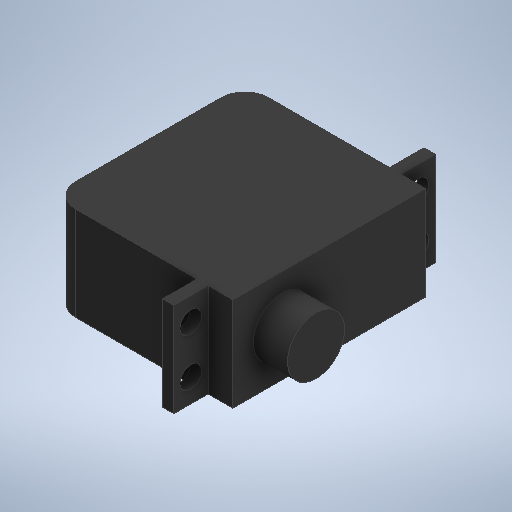
# Autodesk Inventor part: servomoteur_roues
Saved by Autodesk Inventor 2025 (Build 290162000, 162)
## iProperties
Created: 2024-09-04
Part Number: servomoteur_roues
Material: Générique
Document SubType Name: Modeling
Designer: chass
Density: 1 g/cm^3
Appearance: Par défaut
Author: chass
Autodesk Inventor part; units mm, degrees
ref_plane "YZ Plane" through (0, 0, 0) normal (1, 0, 0) x (0, 1, 0)
ref_plane "XZ Plane" through (0, 0, 0) normal (0, 1, 0) x (-1, 0, 0)
ref_plane "XY Plane" through (0, 0, 0) normal (0, 0, 1) x (1, 0, 0)
sketch "Esquisse1" plane through (0, 0, 0) normal (1, 0, 0) x (0, 1, 0)
  line L0 (9.85, 20.25) -> (-9.85, 20.25)
  line L1 (-9.85, 20.25) -> (-9.85, -20.25)
  line L2 (-9.85, -20.25) -> (9.85, -20.25)
  line L3 (9.85, -20.25) -> (9.85, 20.25)
  line L4 (9.85, 20.25) -> (-9.85, -20.25)
  line L5 (-9.85, 20.25) -> (9.85, -20.25)
  point P0 (0, 0)
  point P1 (0, 0)
  point P2 (0, 0)
  dimension "d0" = 19.7
  dimension "d1" = 40.5
  constraints: 12 end point, 2 midpoint, 2 parallel, 1 coincident, 1 horizontal, 1 perpendicular
  measures "d0" distance of L2.end L1.end
  measures "d1" distance of L1.end L0.end
extrude "Extrusion1" add sketch "Esquisse1" along normal blind 38
sketch "Esquisse2" plane through (0, -9.85, -20.25) normal (0, 0, -1) x (-1, 0, 0)
  line L0 (0, 0) -> (-38, 0) projected
  line L1 (0, 19.7) -> (-38, 19.7) projected
  line L2 (-32.8, 0) -> (-30.4, 0)
  line L3 (-30.4, 0) -> (-30.4, 19.7)
  line L4 (-30.4, 19.7) -> (-32.8, 19.7)
  line L5 (-32.8, 19.7) -> (-32.8, 0)
  line L6 (-38, 0) -> (-38, 19.7) projected
  point P0 (0, 9.85)
  dimension "d4" = 5.2
  dimension "d5" = 2.4
  constraints: 8 end point, 2 parallel, 2 point on line, 1 horizontal, 1 perpendicular
  measures "d4" distance between parallel lines of L6 L5
  measures "d5" distance between parallel lines of L5 L3
extrude "Extrusion2" add sketch "Esquisse2" along normal blind 7.2 contours L0 L5 L1 L3
sketch "Esquisse3" plane through (0, -9.85, 20.25) normal (0, 0, 1) x (1, 0, 0)
  line L0 (32.8, 19.7) -> (38, 19.7) projected
  line L1 (32.8, 19.7) -> (30.4, 19.7)
  line L2 (30.4, 19.7) -> (30.4, 0)
  line L3 (30.4, 0) -> (32.8, 0)
  line L4 (32.8, 0) -> (32.8, 19.7)
  point P0 (0, 9.85)
  constraints: 8 end point, 2 parallel, 1 horizontal, 1 perpendicular
extrude "Extrusion3" add sketch "Esquisse3" along normal blind 7.2
sketch "Esquisse4" plane through (32.8, -9.85, 20.25) normal (1, 0, 0) x (0, 0, -1)
  line L0 (40.5, 19.7) -> (0, 19.7) projected
  line L1 (20.25, 19.7) -> (20.25, 0)
  line L2 (0, 0) -> (40.5, 0) projected
  circle A0 centre (-3.6, 14.85) radius 2.25
  line L3 (-7.2, 19.7) -> (-7.2, 0) projected
  line L4 (-7.2, 9.85) -> (47.7, 9.85)
  line L5 (47.7, 0) -> (47.7, 19.7) projected
  circle A1 centre (-3.6, 4.85) radius 2.25
  circle A2 centre (44.1, 14.85) radius 2.25
  circle A3 centre (44.1, 4.85) radius 2.25
  point P0 (20.25, 9.85)
  dimension "d10" = 4.5
  dimension "d11" = 10
  constraints: 4 centre point, 4 end point, 4 midpoint, 3 symmetric about line, 3 other
  measures "d10" diameter of A0
  measures "d11" distance of A0.centre A1.centre
extrude "Extrusion4" cut sketch "Esquisse4" against normal blind 7.2
sketch "Esquisse5" plane through (38, 0, 0) normal (1, 0, 0) x (0, 0, -1)
  circle A0 centre (-10, 0) radius 6
  point P0 (0, 0)
  dimension "d14" = 12
  dimension "d15" = 10
  constraints: 1 centre point
  measures "d14" diameter of A0
  measures "d15" distance of point (0, 0) A0.centre
extrude "Extrusion5" add sketch "Esquisse5" along normal blind 7.2
fillet "Congé1" radius 5 2 edges at (0, 0, 20.25) (0, 0, -20.25)
